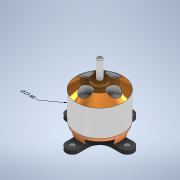
# Autodesk Inventor part: BLDC
Saved by Autodesk Inventor 2020.4 (Build 244396000, 396)
## iProperties
Created: 2021-04-08
Part Number: BLDC
Material: Generic
Document SubType Name: Modeling
Designer: armin
Density: 1 g/cm^3
Appearance: Chrome - Polished
Author: armin
Autodesk Inventor part; units mm, degrees
ref_plane "YZ Plane" through (0, 0, 0) normal (1, 0, 0) x (0, 1, 0)
ref_plane "XZ Plane" through (0, 0, 0) normal (0, 1, 0) x (-1, 0, 0)
ref_plane "XY Plane" through (0, 0, 0) normal (0, 0, 1) x (1, 0, 0)
sketch "Sketch1" plane through (0, 0, 0) normal (0, 1, 0) x (-1, 0, 0)
  line L0 (16.45, 3.75) -> (-16.45, 3.75)
  line L1 (-16.45, 3.75) -> (-16.45, -3.75)
  line L2 (-16.45, -3.75) -> (16.45, -3.75)
  line L3 (16.45, -3.75) -> (16.45, 3.75)
  line L4 (16.45, 3.75) -> (-16.45, -3.75) construction
  line L5 (-16.45, 3.75) -> (16.45, -3.75) construction
  circle A0 centre (16.45, 0) radius 3.75
  circle A1 centre (-16.45, 0) radius 3.75
  line L6 (-20.2, 0) -> (20.2, 0)
  line L7 (3.7, 16.5) -> (-3.7, 16.5)
  line L8 (-3.7, 16.5) -> (-3.7, -16.5)
  line L9 (-3.7, -16.5) -> (3.7, -16.5)
  line L10 (3.7, -16.5) -> (3.7, 16.5)
  line L11 (3.7, 16.5) -> (-3.7, -16.5) construction
  line L12 (-3.7, 16.5) -> (3.7, -16.5) construction
  circle A2 centre (0, 16.5) radius 3.7
  circle A3 centre (0, -16.5) radius 3.7
  line L13 (0, 20.2) -> (0, -20.2)
  circle A4 centre (0, 0) radius 4.95
  line L14 (0, 0) -> (8.1675, 0) construction
  point P0 (3.5002, 3.5002)
  point P1 (5.7753, 5.7753)
  point P2 (-3.7, 3.2882)
  point P3 (-3.7, 3.75)
  point P4 (-16.45, 3.75)
  point P5 (-3.7, -3.75)
  point P6 (-3.7, -3.2882)
  point P7 (-3.2311, 3.75)
  point P8 (3.2311, 3.75)
  point P9 (3.7, 3.75)
  point P10 (3.7, 3.2882)
  point P11 (3.7, -3.2882)
  point P12 (3.7, -3.75)
  point P13 (3.2311, -3.75)
  point P14 (-3.2311, -3.75)
  dimension "d6" = 9.9
  dimension "d0" = 7.5
  dimension "d1" = 40.4
  dimension "d2" = 0
  dimension "d3" = 7.4
  dimension "d4" = 0
  dimension "d5" = 40.4
  constraints: 30 end point, 8 midpoint, 8 point on circle, 4 centre point, 4 horizontal, 4 parallel, 2 perpendicular, 1 coincident, 1 vertical, 3 other
  measures "d0" distance of L1.end L0.end
  measures "d1" distance of L6.start L6.end
  measures "d2" distance from line of point (0, 0) L6
  measures "d3" distance of L9.end L8.end
  measures "d4" distance from line of point (0, 0) L13
  measures "d5" distance of L13.start L13.end
extrude "Extrusion1" add sketch "Sketch1" along normal blind 2.3 contours A0 L6 A4 L10 L0 | A0 L6 L3 | L3 L6 A0 | L10 A4 L0 | L0 A4 L13 A2 L10 | L6 A0 L3 | L3 A0 L6 | A0 L2 L10 A4 L6 | A2 L13 L7 | L7 L13 A2 | A4 L0 L8 A2 L13 | L13 A2 L7 | L7 A2 L13 | L10 A3 L13 A4 L2 | L2 A4 L10 | A4 L8 L0 | A3 L13 L9 | L9 L13 A3 | L8 A4 L6 A1 L0 | L13 A3 L8 L2 A4 | L13 A3 L9 | L9 A3 L13 | A1 L6 L1 | L1 L6 A1 | A4 L8 L2 A1 L6 | A4 L2 L8 | L6 A1 L1 | L1 A1 L6
fillet "Fillet1" radius 7 4 edges at (-3.7, 1.15, 3.75) (-3.7, 1.15, -3.75) (3.7, 1.15, 3.75) (3.7, 1.15, -3.75)
sketch "Sketch2" plane through (0, 2.3, 0) normal (0, 1, 0) x (1, 0, 0)
  arc A0 (-3.7, -16.5) -> (3.7, -16.5) centre (0, -16.5) ccw projected
  circle A1 centre (0, -16.5) radius 1.5
  arc A2 (-16.45, 3.75) -> (-16.45, -3.75) centre (-16.45, 0) ccw projected
  circle A3 centre (-16.45, 0) radius 1.5
  arc A4 (3.7, 16.5) -> (-3.7, 16.5) centre (0, 16.5) ccw projected
  circle A5 centre (0, 16.5) radius 1.5
  arc A6 (16.45, -3.75) -> (16.45, 3.75) centre (16.45, 0) ccw projected
  circle A7 centre (16.45, 0) radius 1.5
  point P0 (0, 0)
  dimension "d12" = 3
  dimension "d13" = 3
  dimension "d14" = 3
  dimension "d15" = 3
  constraints: 4 centre point, 4 coincident
  measures "d12" diameter of A1
  measures "d13" diameter of A3
  measures "d14" diameter of A5
  measures "d15" diameter of A7
extrude "Extrusion2" cut sketch "Sketch2" against normal blind 10
sketch "Sketch3" plane through (0, 0, 0) normal (0, 0, 1) x (1, 0, 0)
  line L0 (0, 0) -> (0, 4.5)
  line L1 (-1.5, 2.3) -> (1.5, 2.3) projected
  line L2 (0, 2.3) -> (-12.5, 2.3)
  line L3 (-16.45, 2.3) -> (-10.7, 2.3) projected
  line L4 (0, 7.3) -> (-13.9, 7.3)
  line L5 (-12.5, 2.3) -> (-13.9, 7.3)
  line L6 (0, 4.5) -> (0, 7.3)
  point P0 (0, 2.3)
  dimension "d18" = 4.5
  dimension "d19" = 12.5
  dimension "d20" = 13.9
  dimension "d21" = 5
  constraints: 10 end point, 2 point on line, 2 vertical, 1 horizontal, 1 midpoint
  measures "d18" distance of L0.start L0.end
  measures "d19" distance of L2.start L2.end
  measures "d20" distance of L4.start L4.end
  measures "d21" distance between parallel lines of L4 L2
revolve "Revolution1" add sketch "Sketch3" angle 360 about axis through (0, 4.5, 0) along (0, 1, 0)
sketch "Sketch4" plane through (-11.9242, 2.3, 3.75) normal (0, -1, 0) x (1, 0, 0)
  arc A0 (8.2242, -14.5) -> (1.2242, -7.5) centre (1.2242, -14.5) ccw projected
  circle A1 centre (1.2242, -14.5) radius 7
  line L0 (8.2242, -15.6898) -> (8.2242, -14.5) projected
  line L1 (8.2242, -14.5) -> (8.2242, -26.697)
  line L2 (8.2242, -26.697) -> (-8.76, -26.697)
  line L3 (-8.76, -26.697) -> (-8.76, -7.5)
  line L4 (1.2242, -7.5) -> (0, -7.5) projected
  line L5 (-8.76, -7.5) -> (1.2242, -7.5)
  point P0 (11.9242, -3.75)
  constraints: 8 end point, 3 perpendicular, 1 centre point, 1 coincident, 1 vertical
extrude "Extrusion3" cut sketch "Sketch4" against normal blind 3
pattern_circular "Circular Pattern1" count 4 over 360 about axis through (0, 0, 0) along (0, 1, 0) of "Extrusion3"
sketch "Sketch5" plane through (0, 7.3, 0) normal (0, 1, 0) x (1, 0, 0)
  circle A0 centre (0, 0) radius 4.95 projected
  circle A1 centre (0, 0) radius 13.9
  constraints: 1 centre point, 1 coincident
extrude "Extrusion4" add sketch "Sketch5" along normal blind 14.8 contours A0 | A1
sketch "Sketch6" plane through (0, 0, 0) normal (0, 0, 1) x (1, 0, 0)
  line L0 (13.9, 22.1) -> (-13.9, 22.1) projected
  line L1 (0, 22.1) -> (-13.9, 22.1)
  line L2 (-13.9, 22.1) -> (-13.9, 23.1)
  line L3 (0, 27.1) -> (-8.5, 27.1)
  line L4 (0, 27.1) -> (0, 22.1)
  line L5 (-8.5, 27.1) -> (-13.9, 23.1)
  point P0 (0, 0)
  dimension "d30" = 1
  dimension "d31" = 8.5
  dimension "d32" = 4
  constraints: 10 end point, 2 horizontal, 1 midpoint, 1 perpendicular, 1 vertical
  measures "d30" distance of L0.end L2.end
  measures "d31" distance of L3.start L3.end
  measures "d32" distance from line of L2.end L3
revolve "Revolution2" add sketch "Sketch6" angle 360 about axis through (0, 27.1, 0) along (0, -1, 0)
sketch "Sketch7" plane through (0, 27.1, 0) normal (0, 1, 0) x (1, 0, 0)
  circle A0 centre (0, 0) radius 8.5 projected
  circle A1 centre (0, 8.4) radius 3.5
  circle A2 centre (0, 0) radius 13.9 projected
  circle A3 centre (-8.4, 0) radius 3.5
  circle A4 centre (0, -8.4) radius 3.5
  circle A5 centre (8.4, 0) radius 3.5
  point P0 (0, 0)
  dimension "d34" = 7
  dimension "d35" = 2
  dimension "d38" = 360
  constraints: 4 centre point, 9 other
  measures "d34" diameter of A1
extrude "Extrusion5" cut sketch "Sketch7" against normal blind 4 contours A0 A5 | A0 A5 | A1 A0 | A0 A1 | A4 A0 | A0 A4 | A3 A0 | A0 A3
sketch "Sketch8" plane through (0, 27.1, 8.4) normal (0, 1, 0) x (1, 0, 0)
  circle A0 centre (0, 8.4) radius 4.5
  dimension "d42" = 9
  constraints: 1 centre point, 1 coincident
  measures "d42" diameter of A0
extrude "Extrusion6" add sketch "Sketch8" along normal blind 1.5
fillet "Fillet2" radius 0.25 1 edges at (-4.5, 28.6, 0)
sketch "Sketch9" plane through (0, 28.6, 0) normal (0, 1, 0) x (1, 0, 0)
  circle A0 centre (0, 0) radius 1.6
  dimension "d46" = 3.2
  constraints: 1 centre point, 1 coincident
  measures "d46" diameter of A0
extrude "Extrusion7" add sketch "Sketch9" along normal blind 11
fillet "Fillet3" radius 0.5 1 edges at (-1.6, 39.6, 0)
body "Solid1"
